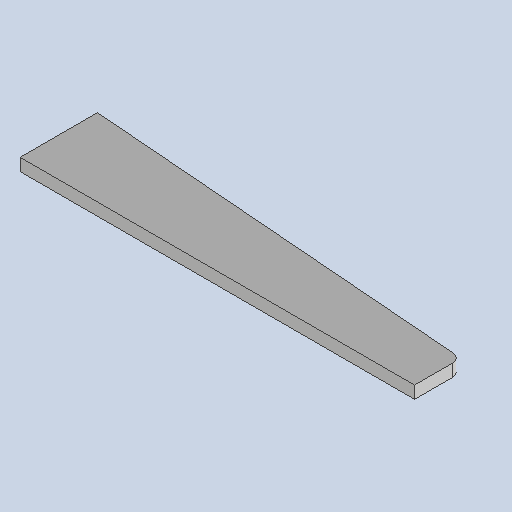
# Autodesk Inventor part: PRS 1614 charging hatch reinf 500mm_D1200 940
Saved by Autodesk Inventor 2026.2 (Build 302298000, 298)
## iProperties
Created: 2025-02-12
Part Number: PRS 1614 charging hatch reinf 500mm_D1200 940
Material: Steel
Document SubType Name: Sheet Metal
Designer: admin
Density: 7.85 g/cm^3
Flat Pattern Width: 4.99208 cm
Flat Pattern Length: 25.7409 cm
Flat Pattern Area: 128.501 cm^2
Sheet Metal Rule: Default_mm
Sheet Metal Width: 49,921 mm
Sheet Metal Length: 257,409 mm
Sheet Metal Area: 12850,059 mm^2
Appearance: Default
Mass: 640.157 g
Surface Area: 250.963 cm^2
Volume: 81.5486 cm^3
Author: pokla
Autodesk Inventor part; units mm, degrees
ref_plane "YZ Plane" through (0, 0, 0) normal (1, 0, 0) x (0, 1, 0)
ref_plane "XZ Plane" through (0, 0, 0) normal (0, 1, 0) x (-1, 0, 0)
ref_plane "XY Plane" through (0, 0, 0) normal (0, 0, 1) x (1, 0, 0)
sketch "Sketch3" plane through (0, 0, 0) normal (0, 0, 1) x (1, 0, 0)
  line L0 (0, 0) -> (300, 0)
  line L1 (300, 0) -> (300, 30)
  line L2 (300, 30) -> (-5.542, 53.9641)
  line L3 (45, 50) -> (45, 0)
  dimension "d11" = 300
  dimension "d12" = 30
  dimension "d13" = 45
  dimension "d14" = 50
  measures "d11" distance of L0.start L0.end
  measures "d12" distance of L0.end L1.end
  measures "d13" distance from line of L0.start L3
  measures "d14" distance of L3.start L3.end
extrude "Plate1" add sketch "Sketch3" along normal mid plane 8
fillet "Corner Round1" radius 6 1 edges at (300, 30, 0)
equation "\"d15\" = Thickness"
equation "\"BendRadius\" = Thickness"
equation "\"BendReliefWidth\" = Thickness"
equation "\"BendReliefDepth\" = 0.5 * Thickness"
equation "\"CornerReliefSize\" = 4 * Thickness"
equation "\"MinimumRemnant\" = 2 * Thickness"
equation "\"TransitionRadius\" = BendRadius"
equation "\"JacobiRadiusSize\" = BendRadius"
equation "\"GapSize\" = Thickness"
equation "\"Thickness\" = 8"
body "Solid2"
